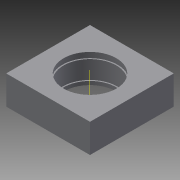
# Autodesk Inventor part: bearing
Saved by Autodesk Inventor 2015 SP1 (Build 190203100, 203)
## iProperties
Created: 2015-04-17
Part Number: bearing
Material: Ogólny
Document SubType Name: Modeling
Designer: Marcin
Density: 1 g/cm^3
Appearance: Domyślna
Author: Marcin
Autodesk Inventor part; units mm, degrees
ref_plane "YZ Plane" through (0, 0, 0) normal (1, 0, 0) x (0, 1, 0)
ref_plane "XZ Plane" through (0, 0, 0) normal (0, 1, 0) x (-1, 0, 0)
ref_plane "XY Plane" through (0, 0, 0) normal (0, 0, 1) x (1, 0, 0)
sketch "Szkic1" plane through (0, 0, 0) normal (0, 0, 1) x (1, 0, 0)
  circle A0 centre (0, 0) radius 11
  line L0 (-17.5, -17.5) -> (17.5, -17.5)
  line L1 (17.5, -17.5) -> (17.5, 17.5)
  line L2 (17.5, 17.5) -> (-17.5, 17.5)
  line L3 (-17.5, 17.5) -> (-17.5, -17.5)
  line L4 (-17.5, -17.5) -> (17.5, 17.5) construction
  line L5 (17.5, -17.5) -> (-17.5, 17.5) construction
  dimension "d0" = 22
  dimension "d1" = 35
  constraints: 12 end point, 2 midpoint, 2 parallel, 2 perpendicular, 1 centre point, 1 coincident, 1 horizontal
  measures "d0" diameter of A0
  measures "d1" distance of L1.end L2.end
extrude "Wyciągnięcie proste1" add sketch "Szkic1" along normal blind 12
sketch "Szkic2" plane through (0, 0, 0) normal (1, 0, 0) x (0, 1, 0)
  line L0 (-11, 12) -> (11, 12) projected
  line L1 (11, 0) -> (-11, 0) projected
  line L2 (-11, 0) -> (-11, 12) projected
  line L3 (-11, 10.6) -> (-11.5, 10.6)
  line L4 (-11.5, 10.6) -> (-11.5, 9.5)
  line L5 (-11.5, 9.5) -> (-11, 9.5)
  line L6 (-11, 9.5) -> (-11, 10.6)
  line L7 (11, 0) -> (11, 12) construction
  line L8 (11, 6) -> (-11, 6) construction
  line L9 (-11, 2.5) -> (-11.5, 2.5)
  line L10 (-11.5, 2.5) -> (-11.5, 1.4)
  line L11 (-11.5, 1.4) -> (-11, 1.4)
  line L12 (-11, 1.4) -> (-11, 2.5)
  line L13 (0, 0) -> (0, 12) construction
  dimension "d4" = 1.1
  dimension "d5" = 0.5
  dimension "d8" = 7
  constraints: 20 end point, 4 parallel, 3 midpoint, 2 equal length, 2 horizontal, 2 perpendicular, 2 point on line, 1 other
  measures "d4" distance of L9.end L10.end
  measures "d5" distance of L9.start L9.end
  measures "d8" distance between parallel lines of L5 L9
revolve "Obrót1" cut sketch "Szkic2" angle 360 about axis through (0, 0, 0) along (0, 0, 1)
sketch "Szkic3" plane through (-17.5, -17.5, 0) normal (0, -1, 0) x (1, 0, 0)
  line L0 (0, 0) -> (35, 0) projected
  line L1 (35, 0) -> (35, 12) projected
  line L2 (0, 12) -> (35, 12) projected
  line L3 (0, 0) -> (0, 12) projected
  line L4 (35, 6) -> (0, 6) construction
  line L5 (0, 12) -> (35, 12) construction
  line L6 (17.5, 12) -> (17.5, 0) construction
  point P0 (31.5, 6)
  point P1 (3.5, 6)
  dimension "d9" = 28
  constraints: 4 end point, 3 midpoint, 2 point on line, 1 symmetric about line, 1 vertical
  measures "d9" distance of point (3.5, 6) point (31.5, 6)
hole "Otwór1" at (14, -17.5, 6) at (-14, -17.5, 6) direction (0, 1, 0) diameter 4 end through all
